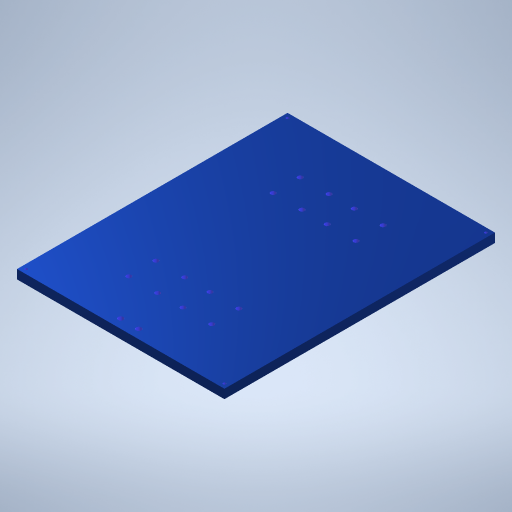
# Autodesk Inventor part: base di lavoro
Saved by Autodesk Inventor 2024 (Build 280153000, 153)
## iProperties
Created: 2023-12-23
Part Number: base di lavoro
Material: Acciaio inox, Austenitico
Document SubType Name: Modeling
Designer: Giorgio
Density: 8 g/cm^3
Appearance: Ottone - Lucidato
Mass: 750 g
Surface Area: 1610 cm^2
Volume: 750 cm^3
Author: Giorgio
Autodesk Inventor part; units mm, degrees
ref_plane "YZ Plane" through (0, 0, 0) normal (1, 0, 0) x (0, 1, 0)
ref_plane "XZ Plane" through (0, 0, 0) normal (0, 1, 0) x (-1, 0, 0)
ref_plane "XY Plane" through (0, 0, 0) normal (0, 0, 1) x (1, 0, 0)
sketch "Schizzo1" plane through (0, 0, 0) normal (0, 1, 0) x (-1, 0, 0)
  line L0 (23.5294, 23.5294) -> (-206.4706, 23.5294)
  line L1 (-206.4706, 23.5294) -> (-206.4706, -276.4706)
  line L2 (-206.4706, -276.4706) -> (23.5294, -276.4706)
  line L3 (23.5294, -276.4706) -> (23.5294, 23.5294)
  circle A0 centre (-45.4706, -31.4706) radius 2.75
  circle A1 centre (-45.4706, -61.4706) radius 2.75
  circle A2 centre (-77.4706, -31.4706) radius 2.75
  circle A3 centre (-77.4706, -61.4706) radius 2.75
  circle A4 centre (-45.4706, -191.4706) radius 2.75
  circle A5 centre (-45.4706, -221.4706) radius 2.75
  circle A6 centre (-77.4706, -191.4706) radius 2.75
  circle A7 centre (-77.4706, -221.4706) radius 2.75
  circle A8 centre (-105.4706, -31.4706) radius 2.75
  circle A9 centre (-105.4706, -61.4706) radius 2.75
  circle A10 centre (-137.4706, -31.4706) radius 2.75
  circle A11 centre (-137.4706, -61.4706) radius 2.75
  circle A12 centre (-105.4706, -191.4706) radius 2.75
  circle A13 centre (-105.4706, -221.4706) radius 2.75
  circle A14 centre (-137.4706, -191.4706) radius 2.75
  circle A15 centre (-137.4706, -221.4706) radius 2.75
  circle A16 centre (-81.4706, 13.5294) radius 3
  circle A17 centre (-101.4706, 13.5294) radius 3
  circle A18 centre (18.5294, 18.5294) radius 1.5
  circle A19 centre (18.5294, -271.4706) radius 1.5
  circle A20 centre (-201.4706, 18.5294) radius 1.5
  circle A21 centre (-201.4706, -271.4706) radius 1.5
  point P0 (0, 0)
  dimension "d0" = 300
  dimension "d1" = 230
  dimension "d4" = 5.5
  dimension "d7" = 30
  dimension "d10" = 32
  dimension "d15" = 160
  dimension "d25" = 60
  dimension "d27" = 55
  dimension "d28" = 69
  dimension "d29" = 6
  dimension "d32" = 20
  dimension "d37" = 10
  dimension "d38" = 105
  dimension "d39" = 3
  dimension "d40" = 5
  dimension "d41" = 5
  dimension "d44" = 290
  dimension "d47" = 220
  constraints: 22 centre point, 8 end point, 5 horizontal, 3 vertical, 2 parallel, 1 perpendicular, 38 other
  measures "d0" distance of L2.end L0.start
  measures "d1" distance of L0.start L0.end
  measures "d4" diameter of A0
  measures "d7" distance of A0.centre A1.centre
  measures "d10" distance of A0.centre A2.centre
  measures "d15" distance of A0.centre A4.centre
  measures "d25" distance of A0.centre A8.centre
  measures "d27" distance from line of L0 A0.centre
  measures "d28" distance from line of L1 A10.centre
  measures "d29" diameter of A16
  measures "d32" distance of A16.centre A17.centre
  measures "d37" distance from line of L0 A17.centre
  measures "d38" distance from line of L3 A16.centre
  measures "d39" diameter of A18
  measures "d40" distance from line of L3 A18.centre
  measures "d41" distance from line of L0 A18.centre
  measures "d44" distance of A18.centre A19.centre
  measures "d47" distance of A18.centre A20.centre
extrude "Estrusione1" add sketch "Schizzo1" along normal blind 10
